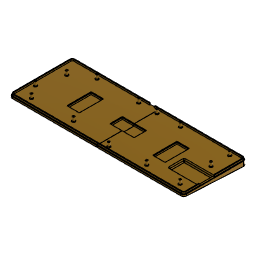
BMMP 2 v94 (Autodesk Fusion 360 design; units mm, degrees)
Autodesk Fusion 360 part; units mm, degrees
sketch "Sketch1" plane through (0, 0, 0) normal (0, 0, 1) x (1, 0, 0)
  line L0 (0, 0) -> (358, 0)
  line L1 (358, 0) -> (358, 129)
  line L2 (358, 129) -> (0, 129)
  line L3 (0, 129) -> (0, 0)
  line L4 (356.6, 127.6) -> (1.4, 127.6)
  line L5 (1.4, 127.6) -> (1.4, 1.4)
  line L6 (1.4, 1.4) -> (356.6, 1.4)
  line L7 (356.6, 1.4) -> (356.6, 127.6)
  line L8 (355, 126) -> (3, 126)
  line L9 (3, 126) -> (3, 3)
  line L10 (3, 3) -> (355, 3)
  line L11 (355, 3) -> (355, 126)
  dimension "d1" = 358
  dimension "d2" = 129
  dimension "d3" = -1.4
  dimension "d4" = -3
  constraint horizontal L0
  constraint vertical L1
  constraint horizontal L2
  constraint vertical L3
  constraint coincident L0.start L3.end
  measures "d1" distance of L0.start L0.end
  measures "d2" distance of L0.start L2.end
extrude "Extrude1" add sketch "Sketch1" along normal blind 2.6 contours L0 L1 L2 L3 | L4 L5 L6 L7 | L8 L9 L10 L11 makes body 1
fillet "Fillet1" radius 6 4 edges at (0, 0, 1.3) (0, 129, 1.3) (358, 129, 1.3) (358, 0, 1.3) on bodies 1
sketch "Sketch2" plane through (0, 0, 2.6) normal (0, 0, 1) x (-1, 0, 0)
  arc A0 (-352, 0) -> (-358, -6) centre (-352, -6) ccw
  line L0 (-358, -6) -> (-358, -123)
  arc A1 (-358, -123) -> (-352, -129) centre (-352, -123) ccw
  line L1 (-352, -129) -> (-6, -129)
  arc A2 (-6, -129) -> (0, -123) centre (-6, -123) ccw
  line L2 (0, -123) -> (0, -6)
  arc A3 (0, -6) -> (-6, 0) centre (-6, -6) ccw
  line L3 (-6, 0) -> (-352, 0)
  line L4 (-356.7, -6) -> (-356.7, -123)
  arc A4 (-356.7, -123) -> (-352, -127.7) centre (-352, -123) ccw
  line L5 (-352, -127.7) -> (-6, -127.7)
  arc A5 (-6, -127.7) -> (-1.3, -123) centre (-6, -123) ccw
  line L6 (-1.3, -123) -> (-1.3, -6)
  arc A6 (-1.3, -6) -> (-6, -1.3) centre (-6, -6) ccw
  line L7 (-6, -1.3) -> (-352, -1.3)
  arc A7 (-352, -1.3) -> (-356.7, -6) centre (-352, -6) ccw
  line L8 (-355, -6) -> (-355, -123)
  arc A8 (-355, -123) -> (-352, -126) centre (-352, -123) ccw
  line L9 (-352, -126) -> (-6, -126)
  arc A9 (-6, -126) -> (-3, -123) centre (-6, -123) ccw
  line L10 (-3, -123) -> (-3, -6)
  arc A10 (-3, -6) -> (-6, -3) centre (-6, -6) ccw
  line L11 (-6, -3) -> (-352, -3)
  arc A11 (-352, -3) -> (-355, -6) centre (-352, -6) ccw
  dimension "d9" = -1.3
  dimension "d10" = -3
extrude "Extrude2" add sketch "Sketch2" along normal blind 3 contours L4 A4 L5 A5 L6 A6 L7 A7 bodies 1
sketch "Sketch3" plane through (0, 129, 0) normal (0, 1, 0) x (-1, 0, 0)
  line L0 (-352, 2.6) -> (-352, 0)
  line L1 (-352, 0) -> (-6, 0)
  line L2 (-6, 0) -> (-6, 2.6)
  line L3 (-6, 2.6) -> (-352, 2.6)
  line L4 (0, 2.6) -> (0, 0) construction
  line L5 (0, 1.3) -> (-161, 1.3) construction
  line L6 (-6, 5.6) -> (-352, 5.6) construction
  line L7 (-161.5, 5.6) -> (-161.5, 2.6) construction
  line L8 (-161.5, 2.6) -> (-171.5, 2.6)
  line L9 (-171.5, 2.6) -> (-171.5, 5.6)
  line L10 (-171.5, 5.6) -> (-161.5, 5.6)
  line L11 (-161.5, 5.6) -> (-161.5, 2.6)
  dimension "d15" = 161
  dimension "d16" = 3
  dimension "d17" = 10
  dimension "d18" = 3
  dimension "d172" = 161.5
  constraint midpoint L4 L5.start
  constraint perpendicular L4 L5
  constraint coincident L6 L7.start
  constraint coincident L3 L7.end
  constraint perpendicular L3 L7
  constraint horizontal L8
  constraint vertical L9
  constraint horizontal L10
  constraint vertical L11
  measures "d15" distance of L5.start L5.end
  measures "d16" distance of L7.start L7.end
  measures "d17" distance of L7.end L8.end
  measures "d18" distance of L7.end L7.start
  measures "d172" distance of L4 L11
extrude "Extrude4" cut sketch "Sketch3" against normal blind 3.5 contours L3 L8 L9 L10 L11 bodies 1
fillet "Fillet2" radius 0.8 2 edges at (171.5, 126.85, 2.6) (161.5, 126.85, 2.6) on bodies 1
sketch "Sketch4" plane through (0, 129, 0) normal (0, 1, 0) x (-1, 0, 0)
  line L0 (-352, 2.6) -> (-352, 0)
  line L1 (-352, 0) -> (-6, 0)
  line L2 (-6, 0) -> (-6, 2.6)
  line L3 (-6, 2.6) -> (-352, 2.6)
  line L4 (-171.5, 3.4) -> (-171.5, 5.6)
  arc A0 (-171.5, 3.4) -> (-170.7, 2.6) centre (-170.7, 3.4) ccw
  arc A1 (-162.3, 2.6) -> (-161.5, 3.4) centre (-162.3, 3.4) ccw
  line L5 (-161.5, 5.6) -> (-161.5, 3.4)
  line L6 (-170.7, 2.6) -> (-162.3, 2.6)
  line L7 (-171.5, 5.6) -> (-161.5, 5.6)
  line L8 (-160, 5.6) -> (-160, 3.4)
  arc A2 (-162.3, 1.1) -> (-160, 3.4) centre (-162.3, 3.4) ccw
  line L9 (-170.7, 1.1) -> (-162.3, 1.1)
  arc A3 (-173, 3.4) -> (-170.7, 1.1) centre (-170.7, 3.4) ccw
  line L10 (-173, 3.4) -> (-173, 5.6)
  dimension "d23" = 1.5
  constraint coincident A0.end L6.start
  constraint coincident A1.start L6.end
  constraint coincident L4.end L7.start
  constraint coincident L5.start L7.end
extrude "Extrude5" cut sketch "Sketch4" against normal blind 1.3 contours L3 L6 A2 L9 A3 bodies 1
fillet "Fillet3" radius 0.3 4 edges at (172.8564, 128.35, 2.6) (160.1436, 128.35, 2.6) (171.5, 126.85, 5.6) (161.5, 126.85, 5.6) on bodies 1
sketch "Sketch6" plane through (0, 0, 2.6) normal (0, 0, 1) x (-1, 0, 0)
  line L0 (-169.7, -127) -> (-161.8, -127)
  line L1 (-161.8, -127) -> (-161.8, -126)
  line L2 (-161.8, -126) -> (-6, -126)
  arc A0 (-6, -126) -> (-3, -123) centre (-6, -123) ccw
  line L3 (-3, -123) -> (-3, -6)
  arc A1 (-3, -6) -> (-6, -3) centre (-6, -6) ccw
  line L4 (-6, -3) -> (-351, -3)
  arc A2 (-351, -3) -> (-354, -6) centre (-351, -6) ccw
  line L5 (-354, -6) -> (-354, -123)
  arc A3 (-354, -123) -> (-351, -126) centre (-351, -123) ccw
  line L6 (-351, -126) -> (-169.7, -126)
  line L7 (-169.7, -126) -> (-169.7, -127)
  line L8 (-351, 0) -> (-351, -35) construction
  line L9 (-357, -6) -> (-357, -123) construction
  line L10 (-351, -35) -> (-357, -35) construction
  line L11 (-357, -35) -> (-294, -35)
  line L12 (-294, -35) -> (-294, -65)
  line L13 (-294, -65) -> (-357, -65)
  line L14 (-357, -65) -> (-357, -35)
  line L15 (-357, -50) -> (-353.5, -50) construction
  line L16 (-353.5, -50) -> (-353.5237, -35)
  line L17 (-353.5, -50) -> (-353.5, -65)
  line L18 (-170.7, -127.7) -> (-162.3, -127.7)
  line L19 (-162.3, -127.7) -> (-162.3, -126)
  line L20 (-162.3, -126) -> (-6, -126)
  arc A4 (-6, -126) -> (-3, -123) centre (-6, -123) ccw
  line L21 (-3, -123) -> (-3, -6)
  arc A5 (-3, -6) -> (-6, -3) centre (-6, -6) ccw
  line L22 (-6, -3) -> (-352, -3)
  arc A6 (-352, -3) -> (-355, -6) centre (-352, -6) ccw
  line L23 (-355, -6) -> (-355, -123)
  arc A7 (-355, -123) -> (-352, -126) centre (-352, -123) ccw
  line L24 (-352, -126) -> (-170.7, -126)
  line L25 (-170.7, -126) -> (-170.7, -127.7)
  point P0 (-351, 0)
  dimension "d57" = 35
  dimension "d58" = 63
  dimension "d59" = 30
  dimension "d62" = 3.5
  constraint coincident P0 L8.start
  constraint vertical L8
  constraint coincident L9 L10.end
  constraint perpendicular L8 L10
  constraint horizontal L11
  constraint vertical L12
  constraint horizontal L13
  constraint vertical L14
  constraint midpoint L14 L15.start
  constraint perpendicular L5 L15
  constraint coincident L11 L16.end
  constraint coincident L13 L17.end
  measures "d57" distance of P0 L8.end
  measures "d58" distance of L10.end L11.end
  measures "d59" distance of L10.end L13.end
  measures "d62" distance of L15.start L15.end
extrude "Extrude7" cut sketch "Sketch6" along normal blind 5 contours L5 L11 L13 L23 | L5 L11 L13 L16 L17 | L11 L12 L13 L16 L17 | L11 L13 L14 L23 bodies 1
extrude "Extrude8" add 1 faces at (236.6667, 43, 0) along direction (0, 0, -1) blind 2 on bodies 1 bodies 1
draft "Draft1" angle 3 neutral plane through (6, 0, 0) pull (0, -1, 0) 1 faces at (236.6667, 43, -2) on bodies 1
extrude "Extrude9" cut sketch "Sketch6" against normal blind 6 contours L5 L11 L13 L16 L17 | L11 L12 L13 L16 L17 bodies 1
fillet "Fillet4" radius 1 2 edges at (294, 65, -0.4) (294, 35, -0.4) on bodies 1
fillet "Fillet5" radius 2 5 edges at (324.5, 35, 2.6) (294.2929, 35.2929, 2.6) (294, 50, 2.6) (294.2929, 64.7071, 2.6) (324.5, 65, 2.6) on bodies 1
fillet "Fillet6" radius 1 2 edges at (355.85, 65, 5.6) (355.85, 35, 5.6) on bodies 1
fillet "Fillet7" radius 0.5 2 edges at (355.85, 35, 2.6) (355.85, 65, 2.6) on bodies 1
fillet "Fillet8" radius 0.5 14 edges at (0, 64.5, 2.6) (1.7574, 127.2426, 2.6) (82.9721, 129, 2.6) (160.1053, 129, 2.5531) (161.0647, 129, 1.4599) (166.5, 129, 1.1) (171.9353, 129, 1.4599) (172.8947, 129, 2.5531) (262.5279, 129, 2.6) (356.2426, 127.2426, 2.6) (358, 64.5, 2.6) (356.2426, 1.7574, 2.6) (179, 0, 2.6) (1.7574, 1.7574, 2.6) on bodies 1
chamfer "Chamfer2" distance 1 angle 45 8 edges at (1.7574, 1.7574, -2.0921) (0, 64.5, -5.3803) (1.7574, 127.2426, -8.6685) (179, 129, -8.7606) (356.2426, 127.2426, -8.6685) (358, 64.5, -5.3803) (356.2426, 1.7574, -2.0921) (179, 0, -2) on bodies 1
sketch "Sketch8" plane through (0, 0, 2.6) normal (0, 0, 1) x (-1, 0, 0)
  line L0 (-295, -67) -> (-354, -67)
  line L1 (-355, -64.5) -> (-355, -123)
  arc A0 (-355, -123) -> (-352, -126) centre (-352, -123) ccw
  line L2 (-352, -126) -> (-170.7, -126)
  line L3 (-170.7, -126) -> (-170.7, -127.7)
  line L4 (-162.3, -127.7) -> (-162.3, -126)
  line L5 (-162.3, -126) -> (-6, -126)
  arc A1 (-6, -126) -> (-3, -123) centre (-6, -123) ccw
  line L6 (-3, -123) -> (-3, -6)
  arc A2 (-3, -6) -> (-6, -3) centre (-6, -6) ccw
  line L7 (-6, -3) -> (-352, -3)
  arc A3 (-352, -3) -> (-355, -6) centre (-352, -6) ccw
  line L8 (-355, -6) -> (-355, -35.5)
  line L9 (-354, -33) -> (-295, -33)
  arc A4 (-292, -36) -> (-295, -33) centre (-295, -36) ccw
  line L10 (-292, -36) -> (-292, -64)
  arc A5 (-295, -67) -> (-292, -64) centre (-295, -64) ccw
  line L11 (-6, -3) -> (-3, -3) construction
  line L12 (-3, -3) -> (-3, -6) construction
  line L13 (-355, -123) -> (-355, -126) construction
  line L14 (-355, -126) -> (-352, -126) construction
  line L15 (-355, -126) -> (-3, -126) construction
  line L16 (-3, -126) -> (-3, -3) construction
  line L17 (-3, -3) -> (-355, -3) construction
  line L18 (-355, -3) -> (-355, -126) construction
  line L19 (0, 0) -> (-357, 0)
  line L20 (-357, 0) -> (-357, -129)
  line L21 (-357, -129) -> (0, -129)
  line L22 (0, -129) -> (0, 0)
  line L23 (0, 0) -> (-28.5, 0) construction
  line L24 (-28.5, 0) -> (-28.5, -16.5) construction
  circle A6 centre (-28.5, -16.5) radius 0.9
  circle A7 centre (-28.5, -16.5) radius 2.25
  line L25 (-3, -3) -> (-14, -3) construction
  line L26 (0, 0) -> (-10.3, 0) construction
  line L27 (-10.3, 0) -> (-10.3, -43) construction
  circle A8 centre (-10.3, -43) radius 0.9
  circle A9 centre (-10.3, -43) radius 2.25
  line L28 (0, -129) -> (-23.5, -129) construction
  line L29 (-23.5, -129) -> (-23.5, -94) construction
  circle A10 centre (-23.5, -94) radius 0.9
  circle A11 centre (-23.5, -94) radius 2.25
  line L30 (0, -129) -> (-2, -129) construction
  line L31 (0, -129) -> (-61.5, -129) construction
  line L32 (-61.5, -129) -> (-61.5, -118.5) construction
  circle A12 centre (-61.5, -118.5) radius 0.9
  circle A13 centre (-61.5, -118.5) radius 2.25
  line L33 (0, -129) -> (-147, -129) construction
  line L34 (-147, -129) -> (-147, -118.5) construction
  circle A14 centre (-147, -118.5) radius 0.9
  circle A15 centre (-147, -118.5) radius 2.25
  line L35 (-170.7, -129) -> (-162.3, -129) construction
  line L36 (-166.5, -129) -> (-166.5, -113) construction
  line L37 (-173.0558, -127.7) -> (-352, -127.7)
  line L38 (-147, -118.5) -> (-184.7, -118.5) construction
  circle A16 centre (-184.7, -118.5) radius 0.9
  circle A17 centre (-184.7, -118.5) radius 2.25
  line L39 (0, 0) -> (-112.5, 0) construction
  line L40 (-112.5, 0) -> (-112.5, -19) construction
  circle A18 centre (-112.5, -19) radius 0.9
  circle A19 centre (-112.5, -19) radius 2.25
  line L41 (-357, 0) -> (-194, 0) construction
  line L42 (-194, 0) -> (-194, -10) construction
  circle A20 centre (-194, -10) radius 0.9
  circle A21 centre (-194, -10) radius 2.25
  line L43 (-357, 0) -> (-334.2, 0) construction
  line L44 (-334.2, 0) -> (-334.2, -16.4) construction
  circle A22 centre (-334.2, -16.4) radius 0.9
  circle A23 centre (-334.2, -16.4) radius 2.25
  line L45 (-334.2, 0) -> (-334.2, -80) construction
  circle A24 centre (-334.2, -80) radius 0.9
  circle A25 centre (-334.2, -80) radius 2.25
  line L46 (-334.2, -80) -> (-334.2, -129) construction
  line L47 (-334.2, -129) -> (-334.2, -118.5) construction
  circle A26 centre (-334.2, -118.5) radius 0.9
  circle A27 centre (-334.2, -118.5) radius 2.25
  line L48 (-357, -129) -> (-233, -129) construction
  line L49 (-233, -129) -> (-233, -118.5) construction
  circle A28 centre (-233, -118.5) radius 0.9
  circle A29 centre (-233, -118.5) radius 2.25
  line L50 (-357, 0) -> (-266, 0) construction
  line L51 (-266, 0) -> (-266, -16) construction
  circle A30 centre (-266, -16) radius 0.9
  circle A31 centre (-266, -16) radius 2.25
  line L52 (-352, -128.5) -> (-173.0558, -128.5)
  line L53 (-173.0558, -128.5) -> (-173.0558, -127.7)
  arc A32 (-356.7, -123) -> (-352, -127.7) centre (-352, -123) ccw
  line L54 (-356.7, -123) -> (-356.7, -64.5)
  line L55 (-356.7, -64.5) -> (-355, -64.5)
  line L56 (-170.7, -127.7) -> (-162.3, -127.7)
  line L57 (-355, -35.5) -> (-356.7, -35.5)
  line L58 (-356.7, -35.5) -> (-356.7, -6)
  arc A33 (-352, -1.3) -> (-356.7, -6) centre (-352, -6) ccw
  line L59 (-352, -1.3) -> (-6, -1.3)
  arc A34 (-1.3, -6) -> (-6, -1.3) centre (-6, -6) ccw
  line L60 (-1.3, -6) -> (-1.3, -123)
  arc A35 (-6, -127.7) -> (-1.3, -123) centre (-6, -123) ccw
  line L61 (-6, -127.7) -> (-159.9442, -127.7)
  line L62 (-159.9442, -127.7) -> (-159.9442, -128.5)
  line L63 (-159.9442, -128.5) -> (-6, -128.5)
  arc A36 (-6, -128.5) -> (-0.5, -123) centre (-6, -123) ccw
  line L64 (-0.5, -123) -> (-0.5, -6)
  arc A37 (-0.5, -6) -> (-6, -0.5) centre (-6, -6) ccw
  line L65 (-6, -0.5) -> (-352, -0.5)
  arc A38 (-352, -0.5) -> (-357.5, -6) centre (-352, -6) ccw
  line L66 (-357.5, -6) -> (-357.5, -123)
  arc A39 (-357.5, -123) -> (-352, -128.5) centre (-352, -123) ccw
  line L67 (-354, -67) -> (-354, -33)
  dimension "d85" = 28.5
  dimension "d86" = 16.5
  dimension "d87" = 1.8
  dimension "d88" = 4.5
  dimension "d93" = 10.3
  dimension "d94" = 43
  dimension "d95" = 1.8
  dimension "d96" = 4.5
  dimension "d97" = 23.5
  dimension "d98" = 35
  dimension "d99" = 1.8
  dimension "d100" = 4.5
  dimension "d101" = 61.5
  dimension "d102" = 10.5
  dimension "d103" = 1.8
  dimension "d104" = 4.5
  dimension "d108" = 147
  dimension "d109" = 10.5
  dimension "d110" = 1.8
  dimension "d111" = 4.5
  dimension "d112" = 37.7
  dimension "d113" = 1.8
  dimension "d114" = 4.5
  dimension "d115" = 112.5
  dimension "d116" = 19
  dimension "d117" = 1.8
  dimension "d118" = 4.5
  dimension "d119" = 163
  dimension "d120" = 10
  dimension "d121" = 1.8
  dimension "d122" = 4.5
  dimension "d123" = 22.8
  dimension "d124" = 16.4
  dimension "d125" = 1.8
  dimension "d126" = 4.5
  dimension "d127" = 80
  dimension "d128" = 1.8
  dimension "d129" = 4.5
  dimension "d130" = 10.5
  dimension "d131" = 1.8
  dimension "d132" = 4.5
  dimension "d133" = 124
  dimension "d134" = 10.5
  dimension "d135" = 1.8
  dimension "d136" = 4.5
  dimension "d137" = 91
  dimension "d138" = 16
  dimension "d139" = 1.8
  dimension "d140" = 4.5
  constraint coincident A2.end L7.start
  constraint tangent A2 L11
  constraint coincident L6.end A2.start
  constraint tangent A2 L12
  constraint coincident L1.end A0.start
  constraint tangent A0 L13
  constraint coincident A0.end L2.start
  constraint tangent A0 L14
  constraint horizontal L15
  constraint vertical L16
  constraint horizontal L17
  constraint vertical L18
  constraint horizontal L19
  constraint vertical L20
  constraint horizontal L21
  constraint vertical L22
  constraint coincident L19.start L22.end
  constraint coincident L19 L23.end
  constraint perpendicular L23 L24
  constraint coincident L24.end A6.centre
  constraint concentric A6 A7
  constraint coincident L7 L25.end
  constraint coincident L23 L26.end
  constraint perpendicular L19 L27
  constraint coincident L27.end A8.centre
  constraint coincident L21 L28.end
  constraint perpendicular L5 L29
  constraint coincident L29.end A10.centre
  constraint concentric A10 A11
  constraint coincident L28 L30.end
  constraint coincident L21 L31.end
  constraint perpendicular L15 L32
  constraint coincident L32.end A12.centre
  constraint concentric A12 A13
  constraint horizontal L33
  constraint perpendicular L15 L34
  constraint coincident L34.end A14.centre
  constraint midpoint L35 L36.start
  constraint perpendicular L15 L36
  constraint parallel L15 L38
  constraint coincident L38.end A16.centre
  constraint concentric A16 A17
  constraint coincident L19 L39.end
  constraint perpendicular L19 L40
  constraint coincident L40.end A18.centre
  constraint concentric A18 A19
  constraint perpendicular L20 L41
  constraint perpendicular L21 L42
  constraint coincident L42.end A20.centre
  constraint concentric A20 A21
  constraint perpendicular L20 L43
  constraint perpendicular L41 L44
  constraint coincident L44.end A22.centre
  constraint concentric A22 A23
  constraint perpendicular L41 L45
  constraint coincident L45.end A24.centre
  constraint concentric A24 A25
  constraint vertical L46
  constraint coincident L21 L46.end
  constraint perpendicular L15 L47
  constraint coincident L47.end A26.centre
  constraint concentric A26 A27
  constraint horizontal L48
  constraint vertical L49
  constraint coincident L49.end A28.centre
  constraint concentric A28 A29
  constraint horizontal L50
  constraint perpendicular L17 L51
  constraint coincident L51.end A30.centre
  constraint concentric A30 A31
  measures "d85" distance of L19.start L23.end
  measures "d86" distance of L23.end L24.end
  measures "d87" diameter of A6
  measures "d88" diameter of A7
  measures "d93" distance of L19.start L26.end
  measures "d94" distance of L26.end L27.end
  measures "d95" diameter of A8
  measures "d96" diameter of A9
  measures "d97" distance of L21.end L28.end
  measures "d98" distance of L28.end L29.end
  measures "d99" diameter of A10
  measures "d100" diameter of A11
  measures "d101" distance of L21.end L31.end
  measures "d102" distance of L31.end L32.end
  measures "d103" diameter of A12
  measures "d104" diameter of A13
  measures "d108" distance of L21.end L33.end
  measures "d109" distance of L33.end L34.end
  measures "d110" diameter of A14
  measures "d111" diameter of A15
  measures "d112" distance of L34.end L38.end
  measures "d113" diameter of A16
  measures "d114" diameter of A17
  measures "d115" distance of L19.start L39.end
  measures "d116" distance of L39.end L40.end
  measures "d117" diameter of A18
  measures "d118" diameter of A19
  measures "d119" distance of L19.end L41.end
  measures "d120" distance of L41.end L42.end
  measures "d121" diameter of A20
  measures "d122" diameter of A21
  measures "d123" distance of L19.end L43.end
  measures "d124" distance of L43.end L44.end
  measures "d125" diameter of A22
  measures "d126" diameter of A23
  measures "d127" distance of L43.end L45.end
  measures "d128" diameter of A24
  measures "d129" diameter of A25
  measures "d130" distance of L46.end L47.end
  measures "d131" diameter of A26
  measures "d132" diameter of A27
  measures "d133" distance of L20.end L48.end
  measures "d134" distance of L48.end L49.end
  measures "d135" diameter of A28
  measures "d136" diameter of A29
  measures "d137" distance of L19.end L50.end
  measures "d138" distance of L50.end L51.end
  measures "d139" diameter of A30
  measures "d140" diameter of A31
extrude "Extrude10" add sketch "Sketch8" along normal blind 8.5 contours A7 | A9 | A11 | A13 | A15 | A17 | A19 | A21 | A23 | A25 | A27 | A29 | A31 bodies 1
chamfer "Chamfer3" distance 1 angle 45 13 edges at (30.5977, 15.6864, 2.6) (12.3977, 42.1864, 2.6) (25.5977, 93.1864, 2.6) (63.5977, 117.6864, 2.6) (149.0977, 117.6864, 2.6) (114.5977, 18.1864, 2.6) (186.7977, 117.6864, 2.6) (196.0977, 9.1864, 2.6) (336.2977, 15.5864, 2.6) (336.2977, 79.1864, 2.6) (336.2977, 117.6864, 2.6) (235.0977, 117.6864, 2.6) (268.0977, 15.1864, 2.6) on bodies 1
sketch "Sketch9" plane through (0, 0, 2.6) normal (0, 0, 1) x (-1, 0, 0)
  circle A0 centre (-233, -118.5) radius 3.25
  circle A1 centre (-194, -10) radius 3.25
  circle A2 centre (-112.5, -19) radius 3.25
  circle A3 centre (-61.5, -118.5) radius 3.25
  circle A4 centre (-10.3, -43) radius 3.25
  line L0 (-295, -67) -> (-354, -67)
  line L1 (-355, -64.5) -> (-355, -123)
  arc A5 (-355, -123) -> (-352, -126) centre (-352, -123) ccw
  line L2 (-352, -126) -> (-170.7, -126)
  line L3 (-170.7, -126) -> (-170.7, -127.7)
  line L4 (-173.0558, -127.7) -> (-352, -127.7)
  line L5 (-162.3, -127.7) -> (-162.3, -126)
  line L6 (-162.3, -126) -> (-6, -126)
  arc A6 (-6, -126) -> (-3, -123) centre (-6, -123) ccw
  line L7 (-3, -123) -> (-3, -6)
  arc A7 (-3, -6) -> (-6, -3) centre (-6, -6) ccw
  line L8 (-6, -3) -> (-352, -3)
  arc A8 (-352, -3) -> (-355, -6) centre (-352, -6) ccw
  line L9 (-355, -6) -> (-355, -35.5)
  line L10 (-354, -33) -> (-295, -33)
  arc A9 (-292, -36) -> (-295, -33) centre (-295, -36) ccw
  line L11 (-292, -36) -> (-292, -64)
  arc A10 (-295, -67) -> (-292, -64) centre (-295, -64) ccw
  circle A11 centre (-28.5, -16.5) radius 3.25
  circle A12 centre (-23.5, -94) radius 3.25
  circle A13 centre (-147, -118.5) radius 3.25
  circle A14 centre (-184.7, -118.5) radius 3.25
  circle A15 centre (-334.2, -16.4) radius 3.25
  circle A16 centre (-334.2, -118.5) radius 3.25
  circle A17 centre (-266, -16) radius 3.25
  line L12 (-179, -3) -> (-179, -150) construction
  circle A18 centre (-334.2, -80) radius 3.25
  line L13 (-352, -128.5) -> (-173.0558, -128.5)
  line L14 (-173.0558, -128.5) -> (-173.0558, -127.7)
  arc A19 (-356.7, -123) -> (-352, -127.7) centre (-352, -123) ccw
  line L15 (-356.7, -123) -> (-356.7, -64.5)
  line L16 (-356.7, -64.5) -> (-355, -64.5)
  line L17 (-355, -35.5) -> (-356.7, -35.5)
  line L18 (-356.7, -35.5) -> (-356.7, -6)
  arc A20 (-352, -1.3) -> (-356.7, -6) centre (-352, -6) ccw
  line L19 (-352, -1.3) -> (-6, -1.3)
  arc A21 (-1.3, -6) -> (-6, -1.3) centre (-6, -6) ccw
  line L20 (-1.3, -6) -> (-1.3, -123)
  arc A22 (-6, -127.7) -> (-1.3, -123) centre (-6, -123) ccw
  line L21 (-6, -127.7) -> (-159.9442, -127.7)
  line L22 (-159.9442, -127.7) -> (-159.9442, -128.5)
  line L23 (-159.9442, -128.5) -> (-6, -128.5)
  arc A23 (-6, -128.5) -> (-0.5, -123) centre (-6, -123) ccw
  line L24 (-0.5, -123) -> (-0.5, -6)
  arc A24 (-0.5, -6) -> (-6, -0.5) centre (-6, -6) ccw
  line L25 (-6, -0.5) -> (-352, -0.5)
  arc A25 (-352, -0.5) -> (-357.5, -6) centre (-352, -6) ccw
  line L26 (-357.5, -6) -> (-357.5, -123)
  arc A26 (-357.5, -123) -> (-352, -128.5) centre (-352, -123) ccw
  line L27 (-354, -67) -> (-354, -33)
  line L28 (-170.7, -127.7) -> (-162.3, -127.7)
  constraint midpoint L8 L12.start
  constraint perpendicular L8 L12
ref_plane "WorkPlane1" through (179.5, 64.5, 0.3) normal (1, 0, 0) x (0, 1, 0)
split "Split1" by plane through (179.5, 64.5, 0.3) normal (1, 0, 0) bodies 1 makes body 2 at (294.5, 43.3329, -4.271)
extrude "Extrude11" cut 1 faces at (179.5, 85.6671, -1.1694) along direction (-1, 0, 0) blind 0.1 on bodies 1 bodies 1
extrude "Extrude12" cut 1 faces at (179.5, 85.6671, -1.1694) along direction (1, 0, 0) blind 0.1 on bodies 2 bodies 2
fillet "Fillet9" radius 1 10 edges at (179.4, 0, 0.55) (179.4, 0.1464, 2.4536) (179.4, 0.9, 2.6) (179.4, 0.4993, -1.5262) (179.4, 1.3, 4.1) (179.4, 128.5007, -8.2344) (179.4, 128.1, 2.6) (179.4, 128.8536, 2.4536) (179.4, 129, -2.8303) (179.4, 127.7, 4.1) on bodies 1
fillet "Fillet10" radius 1 10 edges at (179.6, 0.4993, -1.5262) (179.6, 0.9, 2.6) (179.6, 0.1464, 2.4536) (179.6, 0, 0.55) (179.6, 1.3, 4.1) (179.6, 128.5007, -8.2344) (179.6, 129, -2.8303) (179.6, 128.8536, 2.4536) (179.6, 128.1, 2.6) (179.6, 127.7, 4.1) on bodies 2
sketch "Sketch10" plane through (0, 0, 2.6) normal (0, 0, 1) x (-1, 0, 0)
  line L0 (-179.4, -3) -> (-179.4, -126)
  line L1 (-179.4, -126) -> (-170.7, -126)
  line L2 (-170.7, -126) -> (-170.7, -127.7)
  line L3 (-170.7, -127.7) -> (-162.3, -127.7)
  line L4 (-162.3, -127.7) -> (-162.3, -126)
  line L5 (-162.3, -126) -> (-6, -126)
  arc A0 (-6, -126) -> (-3, -123) centre (-6, -123) ccw
  line L6 (-3, -123) -> (-3, -6)
  arc A1 (-3, -6) -> (-6, -3) centre (-6, -6) ccw
  line L7 (-6, -3) -> (-179.4, -3)
  circle A2 centre (-112.5, -19) radius 3.25
  circle A3 centre (-61.5, -118.5) radius 3.25
  circle A4 centre (-10.3, -43) radius 3.25
  circle A5 centre (-28.5, -16.5) radius 3.25
  circle A6 centre (-23.5, -94) radius 3.25
  circle A7 centre (-147, -118.5) radius 3.25
  line L8 (-179.4, -64.5) -> (-174.4, -64.5) construction
  line L9 (-174.4, -64.5) -> (-155.5, -64.5) construction
  line L10 (-155.5, -64.5) -> (-155.5, -76.25) construction
  line L11 (-155.5, -76.25) -> (-155.5, -52.75) construction
  line L12 (-155.5, -76.25) -> (-203.3, -76.25)
  line L13 (-203.3, -76.25) -> (-203.3, -52.75)
  line L14 (-203.3, -52.75) -> (-155.5, -52.75)
  line L15 (-155.5, -52.75) -> (-155.5, -76.25)
  line L16 (-179.4, -3) -> (-3.8787, -125.1213) construction
  line L17 (-3.8787, -3.8787) -> (-179.4, -126) construction
  line L18 (-91.0079, -64.5) -> (-91.0079, -88.4) construction
  line L19 (-91.0079, -88.4) -> (-79.2579, -88.4) construction
  line L20 (-79.2579, -88.4) -> (-102.7579, -88.4)
  line L21 (-102.7579, -88.4) -> (-102.7579, -40.6)
  line L22 (-102.7579, -40.6) -> (-79.2579, -40.6)
  line L23 (-79.2579, -40.6) -> (-79.2579, -88.4)
  dimension "d150" = 5
  dimension "d151" = 18.9
  dimension "d152" = 11.75
  dimension "d153" = 23.5
  dimension "d154" = 47.8
  dimension "d155" = 23.5
  dimension "d159" = 23.9
  dimension "d160" = 11.75
  dimension "d167" = 23.5
  dimension "d168" = 47.8
  constraint midpoint L0 L8.start
  constraint perpendicular L0 L8
  constraint perpendicular L0 L9
  constraint perpendicular L9 L10
  constraint perpendicular L9 L11
  constraint horizontal L12
  constraint vertical L13
  constraint horizontal L14
  constraint vertical L15
  constraint coincident L0.start L7.end
  constraint midpoint A0 L16.end
  constraint midpoint A1 L17.start
  constraint coincident L0.end L1.start
  constraint coincident L16 L18.start
  constraint coincident L17 L18.start
  constraint vertical L18
  constraint perpendicular L18 L19
  constraint horizontal L20
  constraint vertical L21
  constraint horizontal L22
  constraint vertical L23
  measures "d150" distance of L8.start L8.end
  measures "d151" distance of L8.end L9.end
  measures "d152" distance of L9.end L10.end
  measures "d153" distance of L10.end L11.end
  measures "d154" distance of L10.end L12.end
  measures "d155" distance of L10.end L11.end
  measures "d159" distance of L18.start L18.end
  measures "d160" distance of L18.end L19.end
  measures "d167" distance of L19.end L20.end
  measures "d168" distance of L19.end L22.end
sketch "Sketch11" plane through (0, 0, 2.6) normal (0, 0, 1) x (-1, 0, 0)
  circle A0 centre (-233, -118.5) radius 3.25
  circle A1 centre (-194, -10) radius 3.25
  line L0 (-179.6, -126) -> (-179.6, -3)
  line L1 (-179.6, -3) -> (-352, -3)
  arc A2 (-352, -3) -> (-355, -6) centre (-352, -6) ccw
  line L2 (-355, -64.5) -> (-355, -123)
  line L3 (-354, -33) -> (-295, -33)
  arc A3 (-292, -36) -> (-295, -33) centre (-295, -36) ccw
  line L4 (-292, -36) -> (-292, -64)
  arc A4 (-295, -67) -> (-292, -64) centre (-295, -64) ccw
  line L5 (-295, -67) -> (-354, -67)
  line L6 (-354, -67) -> (-354, -33)
  arc A5 (-355, -123) -> (-352, -126) centre (-352, -123) ccw
  line L7 (-352, -126) -> (-179.6, -126)
  circle A6 centre (-184.7, -118.5) radius 3.25
  circle A7 centre (-334.2, -16.4) radius 3.25
  circle A8 centre (-334.2, -118.5) radius 3.25
  circle A9 centre (-266, -16) radius 3.25
  line L8 (-179.6, -126) -> (-354.1213, -3.8787) construction
  line L9 (-179.6, -3) -> (-354.1213, -125.1213) construction
  line L10 (-267.4885, -64.5) -> (-279.2385, -64.5) construction
  line L11 (-279.2385, -64.5) -> (-279.2385, -88.4) construction
  line L12 (-279.2385, -88.4) -> (-255.7385, -88.4)
  line L13 (-255.7385, -88.4) -> (-255.7385, -40.6)
  line L14 (-255.7385, -40.6) -> (-279.2385, -40.6)
  line L15 (-279.2385, -40.6) -> (-279.2385, -88.4)
  circle A10 centre (-334.2, -80) radius 3.25
  line L16 (-180.6, -128.5) -> (-180.6, -127.7)
  line L17 (-180.6, -127.7) -> (-352, -127.7)
  arc A11 (-356.7, -123) -> (-352, -127.7) centre (-352, -123) ccw
  line L18 (-356.7, -123) -> (-356.7, -64.5)
  line L19 (-356.7, -64.5) -> (-355, -64.5)
  line L20 (-355, -6) -> (-355, -35.5)
  line L21 (-355, -35.5) -> (-356.7, -35.5)
  line L22 (-356.7, -35.5) -> (-356.7, -6)
  arc A12 (-352, -1.3) -> (-356.7, -6) centre (-352, -6) ccw
  line L23 (-352, -1.3) -> (-180.6, -1.3)
  line L24 (-180.6, -1.3) -> (-180.6, -0.5)
  line L25 (-180.6, -0.5) -> (-352, -0.5)
  arc A13 (-352, -0.5) -> (-357.5, -6) centre (-352, -6) ccw
  line L26 (-357.5, -6) -> (-357.5, -123)
  arc A14 (-357.5, -123) -> (-352, -128.5) centre (-352, -123) ccw
  line L27 (-352, -128.5) -> (-180.6, -128.5)
  dimension "d163" = 11.75
  dimension "d164" = 23.9
  dimension "d165" = 23.5
  dimension "d166" = 47.8
  constraint coincident L0.start L7.end
  constraint midpoint A2 L8.end
  constraint coincident L0.end L1.start
  constraint midpoint A5 L9.end
  constraint coincident L9 L10.start
  constraint coincident L8 L10.start
  constraint horizontal L10
  constraint perpendicular L10 L11
  constraint horizontal L12
  constraint vertical L13
  constraint horizontal L14
  constraint vertical L15
  measures "d163" distance of L10.start L10.end
  measures "d164" distance of L10.end L11.end
  measures "d165" distance of L11.end L12.end
  measures "d166" distance of L11.end L14.end
extrude "Extrude13" cut sketch "Sketch11" sketch "Sketch10" against normal blind 4 contours L12 L13 L14 L15 of sketch 2 contours L0 L12 L14 L15 | L0 L12 L13 L14 | L20 L21 L22 L23 bodies 1 2
chamfer "Chamfer4" distance 1 angle 45 14 edges at (191.45, 76.25, 2.6) (203.3, 64.5, 2.6) (191.45, 52.75, 2.6) (255.7385, 64.5, 2.6) (267.4885, 88.4, 2.6) (279.2385, 64.5, 2.6) (267.4885, 40.6, 2.6) (167.45, 76.25, 2.6) (155.5, 64.5, 2.6) (167.45, 52.75, 2.6) (102.7579, 64.5, 2.6) (91.0079, 40.6, 2.6) (79.2579, 64.5, 2.6) (91.0079, 88.4, 2.6) on bodies 1 2
copy_body "Body->Comp1" bodies 1 removing the originals makes body 3 in component "Left"
copy_body "Body->Comp2" bodies 2 removing the originals makes body 4 in component "Right"
move_body "Move1" bodies 4 to x (1, 0, 0) y (0, 0.99863, 0.052336) z (0, -0.052336, 0.99863) at (0, 0.0113, -3.3777) in component "Right"
sketch "Sketch12" plane through (0, 0, -5.3749) normal (0, 0, -1) x (1, 0, 0)
  ellipse E0 centre (178.4, -126.9144) end of major axis (178.4, -128.293) minor radius 1 (178.4, -128.293) -> (179.4, -126.9144) ccw
  line L0 (179.4, -126.9144) -> (179.4, -2.5687)
  ellipse E1 centre (178.4, -2.5687) end of major axis (178.4, -1.116) minor radius 1 (179.4, -2.5687) -> (178.4, -1.116) ccw
  line L1 (178.4, -1.116) -> (6, -1.116)
  spline S0 degree 3 poles (1.0002, -6.0805) (1.0072, -5.2816) (1.2086, -4.4849) (1.8149, -3.3391) (2.1135, -2.9343) (2.465, -2.5824) (2.8164, -2.2305) (3.2205, -1.9315) (4.3771, -1.3179) (5.1882, -1.116) (6, -1.116) knots -1.562074 -1.562074 -1.562074 -1.562074 -1.083563 -1.083563 -0.785398 -0.785398 -0.785398 -0.487233 -0.487233 0 0 0 0
  spline S1 degree 3 poles (1, -6.1242) (1, -6.117) (1, -6.1097) (1.0001, -6.0951) (1.0001, -6.0878) (1.0002, -6.0805) knots -1.570796 -1.570796 -1.570796 -1.570796 -1.566435 -1.566435 -1.562074 -1.562074 -1.562074 -1.562074
  line L2 (1, -6.1242) -> (1, -123.2324)
  line L3 (1, -123.2848) -> (1, -123.2324)
  spline S2 degree 3 poles (6, -128.293) (5.1912, -128.293) (4.3832, -128.0927) (3.2255, -127.4812) (2.8186, -127.1807) (2.465, -126.8266) (2.1113, -126.4726) (1.8112, -126.065) (1.2002, -124.9052) (1, -124.0953) (1, -123.2848) knots 0 0 0 0 0.485398 0.485398 0.785398 0.785398 0.785398 1.085398 1.085398 1.570796 1.570796 1.570796 1.570796
  line L4 (6, -128.293) -> (178.4, -128.293)
  line L5 (0.0002, -123.2848) -> (6, -129.2407) construction
  line L6 (161.2, -127.2432) -> (6, -127.2432) construction
  line L7 (3.0001, -126.2628) -> (15.0001, -126.2628) construction
  line L8 (15.0001, -126.2628) -> (42.7001, -126.2628)
  line L9 (42.7001, -126.2628) -> (42.7001, -115.5628)
  line L10 (42.7001, -115.5628) -> (15.0001, -115.5628)
  line L11 (15.0001, -115.5628) -> (15.0001, -126.2628)
  line L12 (6, 0.0986) -> (178.4, 0.0986) construction
  line L13 (28.8501, -126.2628) -> (28.8501, 0.0986) construction
  line L14 (0, -6.0718) -> (6, -0.0637) construction
  line L15 (3, -3.0678) -> (15, -3.0678) construction
  line L16 (15, -3.0678) -> (34.7, -3.0678)
  line L17 (34.7, -3.0678) -> (34.7, -8.7678)
  line L18 (34.7, -8.7678) -> (15, -8.7678)
  line L19 (15, -8.7678) -> (15, -3.0678)
  line L20 (179.4, -126.9144) -> (179.6, -126.9144) construction
  line L21 (179.5, -126.9144) -> (179.5, -129.9) construction
  line L22 (316.2999, -126.2628) -> (316.2999, -115.5628)
  line L23 (316.2999, -115.5628) -> (343.9999, -115.5628)
  line L24 (343.9999, -115.5628) -> (343.9999, -126.2628)
  line L25 (343.9999, -126.2628) -> (316.2999, -126.2628)
  line L26 (344, -8.7678) -> (344, -3.0678)
  line L27 (344, -3.0678) -> (324.3, -3.0678)
  line L28 (324.3, -3.0678) -> (324.3, -8.7678)
  line L29 (324.3, -8.7678) -> (344, -8.7678)
  point P0 (0.0002, -123.2848)
  point P1 (6, -129.2407)
  point P2 (0, -6.0718)
  point P3 (6, -0.0637)
  point P4 (179.6, -126.9144)
  dimension "d169" = 12
  dimension "d170" = 27.7
  dimension "d171" = 10.7
  dimension "d173" = 12
  dimension "d174" = 19.7
  dimension "d175" = 5.7
  constraint coincident P0 L5.start
  constraint coincident P1 L5.end
  constraint midpoint L5 L7.start
  constraint parallel L6 L7
  constraint horizontal L8
  constraint vertical L9
  constraint horizontal L10
  constraint vertical L11
  constraint midpoint L8 L13.start
  constraint coincident L12 L13.end
  constraint perpendicular L1 L13
  constraint coincident P2 L14.start
  constraint coincident P3 L14.end
  constraint midpoint L14 L15.start
  constraint parallel L10 L15
  constraint horizontal L16
  constraint vertical L17
  constraint horizontal L18
  constraint vertical L19
  constraint coincident L0.start L20.start
  constraint coincident P4 L20.end
  constraint midpoint L20 L21.start
  constraint perpendicular L20 L21
  constraint symmetric L7.end L21 L24.end
  constraint symmetric L8.end L21 L22.start
  constraint symmetric L9.end L21 L22.end
  constraint symmetric L10.end L21 L23.end
  constraint symmetric L15.end L21 L26.end
  constraint symmetric L16.end L21 L27.end
  constraint symmetric L17.end L21 L28.end
  constraint symmetric L18.end L21 L26.start
  measures "d169" distance of L7.start L7.end
  measures "d170" distance of L7.end L8.end
  measures "d171" distance of L7.end L10.end
  measures "d173" distance of L15.start L15.end
  measures "d174" distance of L15.end L16.end
  measures "d175" distance of L15.end L18.end
extrude "Extrude1'" cut sketch "Sketch12" against normal blind 1 contours L8 L9 L10 L11 | L16 L17 L18 L19 | L22 L23 L24 L25 | L26 L27 L28 L29 sketch seen with x (1, 0, 0) y (0, 0.99863, -0.052336) z (0, 0.052336, 0.99863) at (0, 0.1655, 3.3737) bodies 3 in component "Left"
extrude "Extrude1''" cut sketch "Sketch12" against normal blind 1 contours L8 L9 L10 L11 | L16 L17 L18 L19 | L22 L23 L24 L25 | L26 L27 L28 L29 bodies 4 in component "Right"
move_body "Move1'" bodies 3 to x (1, 0, 0) y (0, 0.99863, -0.052336) z (0, 0.052336, 0.99863) at (0, -0.0215, 3.3785) in component "Left"
move_body "Move2" bodies 4 to x (1, 0, 0) y (0, 0.99863, -0.052336) z (0, 0.052336, 0.99863) at (0, -0.0215, 3.3688) in component "Right"
component "Left" placed x (1, 0, 0) y (0, 0.99863, 0.052336) z (0, -0.052336, 0.99863) at (0, 0.0113, -3.3777)
component "Right" placed x (1, 0, 0) y (0, 1, 0) z (0, 0, 1) at (0, 0, 0)
